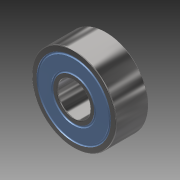
# Autodesk Inventor part: SHU620002RSC3
Saved by Autodesk Inventor 2014 (Build 180170000, 170)
## iProperties
Category: Miscellaneous
Company: Autodesk Inc.
Created: 2013-12-28
Part Number: SHU620002RSC3
Material: Stainless Steel, 440C
Document SubType Name: Modeling
Designer: Autodesk Inc.
Density: 7.75 g/cm^3
Appearance: Steel - Polished
Catalog Web Link: http://www.shusterbearings.com/shopexd.asp?id=98
Vendor: Shuster
Author: Autodesk Inc.
Autodesk Inventor part; units mm, degrees
ref_plane "YZ Plane" through (0, 0, 0) normal (1, 0, 0) x (0, 1, 0)
ref_plane "XZ Plane" through (0, 0, 0) normal (0, 1, 0) x (-1, 0, 0)
sketch "Sketch1" plane through (0, 0, 0) normal (0, 1, 0) x (-1, 0, 0)
  circle A0 centre (0, 0) radius 5
  circle A1 centre (0, 0) radius 13
  dimension "d0" = 10
  dimension "d1" = 26
  constraints: 2 centre point, 2 coincident
  measures "d0" diameter of A0
  measures "d1" diameter of A1
extrude "Extrusion1" add sketch "Sketch1" against normal blind 10
fillet "Fillet1" radius 0.3 4 edges at (13, 0, 0) (13, -10, 0) (5, 0, 0) (5, -10, 0)
sketch "Sketch2" plane through (0, 0, 0) normal (1, 0, 0) x (0, 1, 0)
  line L0 (-10, -12.7) -> (-10, 12.7) projected
  line L1 (-0.3, 13) -> (-9.7, 13) projected
  circle A0 centre (-10, 11.0851) radius 0.3168
  circle A1 centre (-10, 6.5932) radius 0.3168
  line L2 (-11.3512, 0) -> (1.8919, 0) projected
  point P0 (0, 0)
  constraints: 2 centre point, 2 point on line, 1 equal radius
revolve "Revolution1" cut sketch "Sketch2" angle 360 about axis through (0, -10, 0) along (0, 1, 0)
ref_plane "Work Plane1" through (0, -5, 0) normal (0, 1, 0) x (1, 0, 0)
mirror "Mirror1" about plane through (0, -5, 0) normal (0, 1, 0) of "Revolution1"
body "Solid1"
